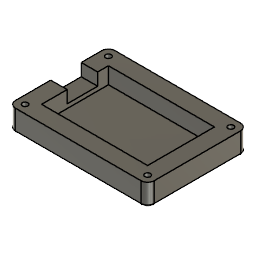
hackpad bottom (Autodesk Fusion 360 design; units mm, degrees)
Autodesk Fusion 360 part; units mm, degrees
sketch "Sketch1" plane through (0, 0, 0) normal (0, 0, 1) x (1, 0, 0) in component "Hackpad"
  line L0 (0, 0) -> (64.4, 0)
  line L1 (64.4, 0) -> (64.4, -40.6)
  line L2 (64.4, -40.6) -> (0, -40.6)
  line L3 (0, -40.6) -> (0, 0)
  line L4 (74.4, -50.6) -> (-10, -50.6)
  line L5 (-10, -50.6) -> (-10, 10)
  line L6 (-10, 10) -> (74.4, 10)
  line L7 (74.4, 10) -> (74.4, -50.6)
  circle A0 centre (-5, 5) radius 1.7
  circle A1 centre (69.4, 5) radius 1.7
  circle A2 centre (69.4, -45.6) radius 1.7
  circle A3 centre (-5, -45.6) radius 1.7
  circle A4 centre (-5, 5) radius 3
  circle A5 centre (69.4, 5) radius 3
  circle A6 centre (69.4, -45.6) radius 3
  circle A7 centre (-5, -45.6) radius 3
  dimension "d1" = 40.6
  dimension "d2" = 64.4
  dimension "d3" = -10
  dimension "d4" = 3.4
  dimension "d5" = 3.4
  dimension "d6" = 3.4
  dimension "d7" = 3.4
  dimension "d8" = 5
  dimension "d9" = 5
  dimension "d10" = 5
  dimension "d11" = 5
  dimension "d12" = 5
  dimension "d13" = 5
  dimension "d14" = 5
  dimension "d15" = 5
  dimension "d16" = 6
  dimension "d17" = 6
  dimension "d18" = 6
  dimension "d19" = 6
  constraint horizontal L0
  constraint vertical L1
  constraint horizontal L2
  constraint vertical L3
  constraint coincident L0.start L3.end
  constraint concentric A0 A4
  constraint concentric A1 A5
  constraint concentric A2 A6
  constraint concentric A3 A7
  measures "d1" distance of L0.start L2.end
  measures "d2" distance of L0.start L0.end
  measures "d4" diameter of A0
  measures "d5" diameter of A1
  measures "d6" diameter of A2
  measures "d7" diameter of A3
  measures "d8" distance of L5 A0.centre
  measures "d9" distance of L6 A0.centre
  measures "d10" distance of L5 A3.centre
  measures "d11" distance of L4 A3.centre
  measures "d12" distance of L7 A2.centre
  measures "d13" distance of L4 A2.centre
  measures "d14" distance of L6 A1.centre
  measures "d15" distance of L7 A1.centre
  measures "d16" diameter of A4
  measures "d17" diameter of A5
  measures "d18" diameter of A6
  measures "d19" diameter of A7
extrude "Extrude1" add sketch "Sketch1" along normal blind 9.9 from surface at 3.1 contours A4 | A5 | A6 | A7 makes body 1 at (70.2125, 7.8879, 9.7) makes body 2 at (70.2125, -42.7121, 9.7) makes body 3 at (-2.0037, 4.8505, 9.7) makes body 4 at (-2.0037, -45.7495, 9.7) in component "Hackpad"
extrude "Extrude2" add sketch "Sketch1" along normal blind 13 contours L4 L5 L6 L7 bodies 1 2 3 4 in component "Hackpad"
extrude "Extrude3" add sketch "Sketch1" along normal blind 3 contours L0 L1 L2 L3 bodies 1 in component "Hackpad"
sketch "Sketch2" plane through (0, 0, 13) normal (0, 0, 1) x (-1, 0, 0) in component "Hackpad"
  circle A0 centre (-69.4, -5) radius 1.7
  circle A1 centre (5, 45.6) radius 1.7
  line L0 (-64.4, 40.6) -> (0, 40.6)
  line L1 (0, 40.6) -> (0, 0)
  line L2 (0, 0) -> (-64.4, 0)
  line L3 (-64.4, 0) -> (-64.4, 40.6)
  line L4 (-74.4, -10) -> (10, -10)
  line L5 (10, -10) -> (10, 50.6)
  line L6 (10, 50.6) -> (-74.4, 50.6)
  line L7 (-74.4, 50.6) -> (-74.4, -10)
  circle A2 centre (-69.4, 45.6) radius 1.7
  circle A3 centre (5, -5) radius 1.7
  line L8 (10, 6.55) -> (0, 6.55)
  line L9 (0, 6.55) -> (0, 25.05)
  line L10 (0, 25.05) -> (10, 25.05)
  line L11 (10, 25.05) -> (10, 6.55)
  line L12 (-74.4, 50.6) -> (10, 50.6)
  dimension "d27" = 18.5
  dimension "d28" = 25.55
  constraint horizontal L8
  constraint vertical L9
  constraint horizontal L10
  constraint vertical L11
  constraint coincident L5 L8.start
  measures "d27" distance of L8.start L10.end
  measures "d28" distance of L10 L12
extrude "Extrude4" cut sketch "Sketch2" against normal blind 7.5 contours L1 L5 L8 L9 L10 L11 bodies 1 in component "Hackpad"
fillet "Fillet1" radius 4 4 edges at (-10, -50.6, 6.5) (74.4, -50.6, 6.5) (74.4, 10, 6.5) (-10, 10, 6.5) on bodies 1 in component "Hackpad"
fillet "Fillet2" radius 1 8 edges at (-8.8284, 8.8284, 0) (32.2, 10, 0) (73.2284, 8.8284, 0) (74.4, -20.3, 0) (73.2284, -49.4284, 0) (32.2, -50.6, 0) (-8.8284, -49.4284, 0) (-10, -20.3, 0) on bodies 1 in component "Hackpad"
component "Hackpad" placed x (1, 0, 0) y (0, 1, 0) z (0, 0, 1) at (0, 0, 0)
equation "d1 = 39.6 mm + 1 mm"
equation "d2 = 63.4 mm + 1 mm"
equation "d28 = 19.8 mm + 5.75 mm"
